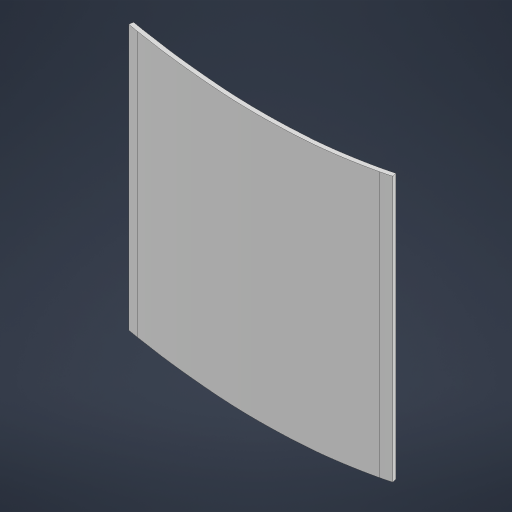
# Autodesk Inventor part: Panele
Saved by Autodesk Inventor 2023 (Build 270158000, 158)
## iProperties
Created: 2023-02-10
Part Number: Panele
Material: Generic
Document SubType Name: Modeling
Designer: szykr
Density: 1 g/cm^3
Appearance: Default
Author: szykr
Autodesk Inventor part; units mm, degrees
ref_plane "YZ Plane" through (0, 0, 0) normal (1, 0, 0) x (0, 1, 0)
ref_plane "XZ Plane" through (0, 0, 0) normal (0, 1, 0) x (-1, 0, 0)
ref_plane "XY Plane" through (0, 0, 0) normal (0, 0, 1) x (1, 0, 0)
sketch "Sketch1" plane through (0, 0, 0) normal (0, 1, 0) x (-1, 0, 0)
  spline S0 degree 3 poles (43.1522, 5.3243) (42.3315, 5.4664) (41.5093, 5.6073) (39.8666, 5.8857) (39.0444, 6.0233) (38.2223, 6.159) knots 0 0 0 0 0.499933 0.499933 1 1 1 1
  spline S1 degree 3 poles (66.2259, 1.043) (62.6029, 1.7785) (58.6834, 2.5166) (51.798, 3.7917) (47.2188, 4.6203) (43.1522, 5.3243) knots 0 0 0 0 1.10907 1.10907 2.509245 2.509245 2.509245 2.509245
  spline S2 degree 3 poles (71.1391, 0.018) (70.321, 0.1929) (69.5028, 0.3659) (67.8628, 0.7083) (67.0477, 0.8762) (66.2259, 1.043) knots 0 0 0 0 0.250983 0.250983 0.502621 0.502621 0.502621 0.502621
  spline S3 degree 3 poles (100.0196, -7.1406) (100.0208, -7.1354) (100.0209, -7.13) (100.019, -7.1179) (100.0165, -7.1114) (100.0075, -7.0943) (99.9988, -7.0838) (99.9675, -7.0518) (99.9354, -7.0292) (99.7974, -6.9442) (99.6273, -6.8698) (98.578, -6.4707) (96.8058, -5.9602) (87.4188, -3.5895) (77.8842, -1.4241) (71.1391, 0.018) knots 0 0 0 0 0.003623 0.003623 0.008208 0.008208 0.01664 0.01664 0.03832 0.03832 0.1102 0.1102 0.407101 0.407101 1 1 1 1
  spline S4 degree 3 poles (88.3221, -6.0834) (91.7402, -6.4934) (94.4085, -6.8236) (97.4322, -7.1281) (98.4156, -7.2175) (99.3319, -7.2475) (99.5896, -7.2498) (99.8412, -7.2231) (99.9048, -7.2123) (99.9684, -7.1892) (99.9857, -7.1811) (100.0039, -7.1666) (100.0088, -7.1618) (100.0159, -7.1515) (100.0184, -7.1463) (100.0196, -7.1406) knots 0 0 0 0 1.032775 1.032775 1.426182 1.426182 1.558102 1.558102 1.606872 1.606872 1.625804 1.625804 1.633391 1.633391 1.640028 1.640028 1.640028 1.640028
  spline S5 degree 3 poles (83.37, -5.5037) (84.1975, -5.5971) (85.0257, -5.6928) (86.6772, -5.8867) (87.4943, -5.9841) (88.3221, -6.0834) knots 0 0 0 0 0.501042 0.501042 1 1 1 1
  spline S6 degree 3 poles (-80.3402, 5.1536) (-83.2822, 4.278) (-86.9469, 2.7724) (-90.9829, 1.0041) (-94.5535, -0.8137) (-97.494, -3.1687) (-98.2105, -3.8005) (-99.1921, -4.921) (-99.5356, -5.4063) (-99.8868, -6.2147) (-99.9775, -6.5471) (-99.996, -7.1728) (-99.9491, -7.4459) (-99.7408, -7.9881) (-99.5798, -8.2401) (-99.0999, -8.8123) (-98.7333, -9.1116) (-97.8214, -9.7276) (-97.0693, -10.1264) (-95.5344, -10.6309) (-94.6795, -10.8081) (-86.0276, -11.9257) (-83.5865, -11.7916) (-79.0114, -11.6226) (-70.8952, -11.1542) (-60.4886, -10.5087) (-55.0368, -10.1095) (-44.8902, -9.0581) (-36.6849, -8.1844) (-26.6949, -7.2523) (-13.6037, -6.0273) (1.2561, -4.8792) (6.6493, -4.6998) (30.6513, -3.7055) (33.9966, -3.3748) (56.1985, -4.0849) (56.7678, -4.1014) (69.2783, -4.2473) (73.4546, -4.385) (83.37, -5.5037) knots 0 0 0 0 0.920867 0.920867 2.748385 2.748385 3.274223 3.274223 3.647653 3.647653 3.885224 3.885224 4.081385 4.081385 4.287479 4.287479 4.599167 4.599167 5.052723 5.052723 5.427905 5.427905 6.514514 6.514514 8.824105 8.824105 12.215959 12.215959 13.039612 13.039612 13.387005 13.387005 13.841738 13.841738 14.651769 14.651769 15.011097 15.011097 15.310395 15.310395 15.310395 15.310395
  spline S7 degree 3 poles (-75.502, 6.4152) (-76.3067, 6.2273) (-77.1275, 6.0275) (-78.7331, 5.6124) (-79.5438, 5.3906) (-80.3402, 5.1536) knots 0 0 0 0 0.500004 0.500004 1 1 1 1
  spline S8 degree 3 poles (38.2223, 6.159) (27.9475, 7.8551) (19.1532, 8.9329) (-7.8876, 11.6415) (-18.2273, 12.0298) (-42.3592, 11.3757) (-48.6068, 10.8186) (-61.3144, 9.3487) (-69.9295, 7.7161) (-75.502, 6.4152) knots 0 0 0 0 3.124155 3.124155 9.518563 9.518563 14.091564 14.091564 23.667143 23.667143 23.667143 23.667143
  spline S9 degree 3 poles (71.16, 0.1157) (76.6898, -1.0665) (83.3896, -2.5841) (91.1027, -4.4231) (94.4588, -5.2395) (97.5341, -6.0864) (98.563, -6.3783) (99.4741, -6.7017) (99.714, -6.7939) (99.9439, -6.915) (100.0045, -6.9522) (100.0735, -7.0152) (100.0907, -7.0376) (100.1097, -7.0737) (100.1154, -7.0895) (100.1227, -7.1305) (100.12, -7.1501) (100.1172, -7.1624) knots 0 0 0 0 1.696424 1.696424 2.44904 2.44904 2.662496 2.662496 2.730748 2.730748 2.757666 2.757666 2.774085 2.774085 2.785515 2.785515 2.802376 2.802376 2.802376 2.802376
  spline S10 degree 3 poles (66.2458, 1.141) (67.0677, 0.9742) (67.8829, 0.8063) (69.5234, 0.4638) (70.3418, 0.2907) (71.16, 0.1157) knots 0 0 0 0 0.251575 0.251575 0.502459 0.502459 0.502459 0.502459
  spline S11 degree 3 poles (43.1692, 5.4229) (47.2367, 4.7187) (51.8267, 3.8881) (58.6927, 2.6166) (62.6216, 1.8767) (66.2458, 1.141) knots 0 0 0 0 1.23838 1.23838 2.219097 2.219097 2.219097 2.219097
  spline S12 degree 3 poles (38.2386, 6.2577) (39.0609, 6.122) (39.8832, 5.9843) (41.5261, 5.7059) (42.3484, 5.5649) (43.1692, 5.4229) knots 0 0 0 0 0.500067 0.500067 1 1 1 1
  spline S13 degree 3 poles (-75.5247, 6.5126) (-72.2701, 7.2724) (-60.0806, 9.9292) (-39.537, 11.624) (-31.0973, 11.8149) (-16.4407, 11.9585) (-7.648, 11.6112) (19.1618, 9.1057) (28.23, 7.9098) (38.2386, 6.2577) knots 0 0 0 0 1.002641 1.002641 1.586612 1.586612 2.736705 2.736705 3.806793 3.806793 3.806793 3.806793
  spline S14 degree 3 poles (-80.3687, 5.2494) (-79.5708, 5.4869) (-78.7587, 5.7091) (-77.1519, 6.1245) (-76.3306, 6.3244) (-75.5247, 6.5126) knots 0 0 0 0 0.499965 0.499965 1 1 1 1
  spline S15 degree 3 poles (83.3587, -5.6031) (75.8338, -4.7541) (71.2171, -4.423) (63.0763, -4.2593) (60.5743, -4.3016) (45.89, -3.876) (40.1735, -3.5496) (26.2872, -3.9476) (23.855, -4.0783) (5.7068, -4.8523) (1.6068, -4.9189) (-14.9038, -6.2524) (-28.7569, -7.5451) (-40.8533, -8.6747) (-44.9578, -9.1707) (-57.2636, -10.422) (-64.8382, -10.9037) (-83.9685, -11.9819) (-84.6152, -11.9986) (-90.0569, -11.4994) (-92.1017, -11.255) (-95.0997, -10.8278) (-95.9036, -10.6544) (-97.3262, -10.0915) (-97.9449, -9.7713) (-98.8418, -9.1537) (-99.205, -8.8504) (-99.7077, -8.2367) (-99.8828, -7.9431) (-100.0757, -7.3344) (-100.1057, -7.0447) (-100.0507, -6.4271) (-99.9566, -6.1154) (-99.6173, -5.3587) (-99.3082, -4.9211) (-98.3779, -3.8124) (-97.5855, -3.1068) (-94.7697, -0.8788) (-91.4921, 0.8379) (-88.0288, 2.4212) (-83.9774, 4.1755) (-80.3687, 5.2494) knots 0 0 0 0 2.271794 2.271794 3.492265 3.492265 4.943094 4.943094 5.554122 5.554122 6.779206 6.779206 7.500678 7.500678 15.370973 15.370973 37.081903 37.081903 69.577181 69.577181 84.528966 84.528966 99.973288 99.973288 111.121624 111.121624 119.002016 119.002016 124.961046 124.961046 130.137791 130.137791 135.773633 135.773633 144.620011 144.620011 161.147321 161.147321 203.473601 203.473601 223.476886 223.476886 223.476886 223.476886
  spline S16 degree 3 poles (88.3102, -6.1827) (87.4831, -6.0835) (86.6655, -5.9861) (85.0141, -5.7922) (84.1861, -5.6964) (83.3587, -5.6031) knots 0 0 0 0 0.249891 0.249891 0.500826 0.500826 0.500826 0.500826
  spline S17 degree 3 poles (100.1172, -7.1624) (100.1146, -7.1743) (100.1092, -7.1916) (100.0867, -7.2256) (100.074, -7.2388) (100.0392, -7.266) (100.0166, -7.2771) (99.9548, -7.302) (99.9026, -7.3136) (99.663, -7.3489) (99.3874, -7.3493) (97.3054, -7.2818) (93.1035, -6.7576) (88.3102, -6.1827) knots 0 0 0 0 0.015283 0.015283 0.027652 0.027652 0.045345 0.045345 0.084745 0.084745 0.209887 0.209887 1 1 1 1
  line L0 (-80.9392, 7.1663) -> (-80.3687, 5.2494)
  line L1 (43.5104, 7.3935) -> (43.1692, 5.4229)
  circle A0 centre (-92.98, -6.2739) radius 1.75
  circle A1 centre (49.02, 0.2394) radius 1.75
  spline S18 degree 3 poles (-80.9392, 7.1663) (-79.301, 7.6531) (-77.6432, 8.071) (-75.9794, 8.4602) knots 0 0 0 0 1 1 1 1
  spline S19 degree 5 poles (-75.9794, 8.4602) (-74.9841, 8.6924) (-73.986, 8.9125) (-72.9867, 9.1274) (-70.3213, 9.6814) (-67.6475, 10.1948) (-65.9747, 10.5) (-62.2039, 11.1542) (-58.4201, 11.728) (-56.3137, 12.0229) (-51.903, 12.577) (-47.4776, 13.0027) (-45.1648, 13.1724) (-40.692, 13.4519) (-36.2141, 13.6384) (-34.0525, 13.7115) (-30.3198, 13.8106) (-26.5863, 13.8639) (-25.0153, 13.8787) (-21.9503, 13.886) (-18.8855, 13.8497) (-17.3918, 13.8206) (-14.287, 13.7365) (-11.184, 13.6044) (-9.5741, 13.5236) (-6.119, 13.3255) (-2.6669, 13.0812) (-0.8235, 12.9387) (3.0583, 12.6193) (6.9368, 12.2612) (8.9736, 12.0665) (12.8257, 11.684) (16.6741, 11.2664) (18.4875, 11.0614) (21.9658, 10.6492) (25.4396, 10.2) (27.1022, 9.9757) (30.3954, 9.5131) (33.6836, 9.0159) (35.3117, 8.7613) (36.9385, 8.4994) (38.5644, 8.231) knots 0 0 0 0 0 0 0.044336 0.044336 0.044336 0.118096 0.118096 0.118096 0.210345 0.210345 0.210345 0.310921 0.310921 0.310921 0.404745 0.404745 0.404745 0.472894 0.472894 0.472894 0.5377 0.5377 0.5377 0.60762 0.60762 0.60762 0.687822 0.687822 0.687822 0.776579 0.776579 0.776579 0.855742 0.855742 0.855742 0.928519 0.928519 0.928519 1 1 1 1 1 1
  spline S20 degree 3 poles (38.5644, 8.231) (40.2142, 7.9587) (41.8627, 7.6788) (43.5104, 7.3935) knots 0 0 0 0 1 1 1 1
  point P0 (0, 0)
  constraints: 4 end point, 9 other
extrude "Extrusion1" add sketch "Sketch1" against normal blind 125 contours S12 S13 S14 L0 S18 S19 S20 L1
body "Solid1"
